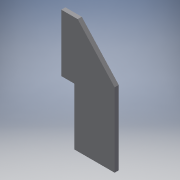
# Autodesk Inventor part: motor mount platform
Saved by Autodesk Inventor 2019 (Build 230136000, 136)
## iProperties
Created: 2018-08-20
Part Number: motor mount platform
Material: Generic
Document SubType Name: Modeling
Designer: kalakuntla1297
Density: 1 g/cm^3
Appearance: Default
Author: kalakuntla1297
Autodesk Inventor part; units mm, degrees
ref_plane "YZ Plane" through (0, 0, 0) normal (1, 0, 0) x (0, 1, 0)
ref_plane "XZ Plane" through (0, 0, 0) normal (0, 1, 0) x (-1, 0, 0)
ref_plane "XY Plane" through (0, 0, 0) normal (0, 0, 1) x (1, 0, 0)
sketch "Sketch1" plane through (0, 0, 0) normal (0, 0, 1) x (1, 0, 0)
  line L0 (0, 0) -> (124.46, 0)
  line L1 (124.46, 0) -> (124.46, 228.6)
  line L2 (124.46, 228.6) -> (0, 228.6)
  line L3 (0, 228.6) -> (0, 0)
  dimension "d0" = 124.46
  dimension "d1" = 228.6
  constraints: 8 end point, 2 parallel, 1 horizontal, 1 perpendicular
  measures "d0" distance of L1.end L2.end
  measures "d1" distance of L0.end L1.end
extrude "Extrusion1" add sketch "Sketch1" along normal blind 12.7
sketch "Sketch3" plane through (0, 0, 12.7) normal (0, 0, 1) x (1, 0, 0)
  line L0 (124.46, 0) -> (124.46, 228.6) projected
  line L1 (124.46, 228.6) -> (10.16, 354.1146)
  line L2 (10.16, 354.1146) -> (10.16, 228.6)
  line L3 (10.16, 228.6) -> (124.46, 228.6)
  point P0 (0, 0)
  constraints: 6 end point, 1 parallel, 1 perpendicular
extrude "Extrusion2" add sketch "Sketch3" against normal blind 12.7
sketch "Sketch4" plane through (0, 0, 0) normal (0, 0, -1) x (-1, 0, 0)
  line L0 (-10.16, 354.1146) -> (40.64, 354.1146)
  line L1 (40.64, 354.1146) -> (40.64, 176.3146)
  line L2 (40.64, 176.3146) -> (-10.16, 176.3146)
  line L3 (-10.16, 176.3146) -> (-10.16, 354.1146)
  point P0 (0, 0)
  point P1 (-10.16, 354.1146)
  dimension "d6" = 50.8
  dimension "d7" = 177.8
  constraints: 8 end point, 2 parallel, 1 horizontal, 1 perpendicular, 1 point on line
  measures "d6" distance of L1.end L2.end
  measures "d7" distance of L0.end L1.end
extrude "Extrusion3" add sketch "Sketch4" against normal blind 12.7
body "Solid1"
